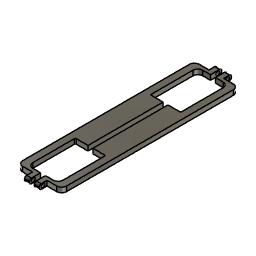
_Arm limb 1.2eed6a4d-bf02-4668-9319-046f86bff51b (Autodesk Fusion 360 design; units mm, degrees)
Autodesk Fusion 360 part; units mm, degrees
sketch "Sketch1" plane through (0, 0, 0) normal (0, 0, 1) x (1, 0, 0)
  line L0 (20, -90.5) -> (-20, -90.5)
  line L1 (-20, -90.5) -> (-20, 90.5)
  line L2 (-20, 90.5) -> (20, 90.5)
  line L3 (20, 90.5) -> (20, -90.5)
  line L4 (20, -90.5) -> (-20, 90.5) construction
  line L5 (-20, -90.5) -> (20, 90.5) construction
  dimension "d1" = 40
  dimension "d2" = 181
  constraint horizontal L0
  constraint perpendicular L0 L1
  constraint parallel L0 L2
  constraint parallel L1 L3
  constraint coincident L4 origin
  constraint coincident L5 origin
  measures "d1" distance of L1.end L2.end
  measures "d2" distance of L0.end L1.end
extrude "Extrude1" add sketch "Sketch1" along normal blind 5 makes body 1
sketch "Sketch2" plane through (0, 0, 5) normal (0, 0, 1) x (-1, 0, 0)
  line L0 (-20, -90.5) -> (20, -90.5)
  line L1 (20, -90.5) -> (20, 90.5)
  line L2 (20, 90.5) -> (-20, 90.5)
  line L3 (-20, 90.5) -> (-20, -90.5)
  line L4 (13, -38.45) -> (-13, -38.45)
  line L5 (-13, -38.45) -> (-13, -87.05)
  line L6 (-13, -87.05) -> (13, -87.05)
  line L7 (13, -87.05) -> (13, -38.45)
  line L8 (13, -38.45) -> (-13, -87.05) construction
  line L9 (-13, -38.45) -> (13, -87.05) construction
  line L10 (-13, 87.05) -> (13, 87.05)
  line L11 (13, 87.05) -> (13, 38.45)
  line L12 (13, 38.45) -> (-13, 38.45)
  line L13 (-13, 38.45) -> (-13, 87.05)
  line L14 (-13, 87.05) -> (13, 38.45) construction
  line L15 (13, 87.05) -> (-13, 38.45) construction
  point P0 (0, -62.75)
  point P1 (0, 62.75)
  dimension "d5" = 26
  dimension "d6" = 48.6
  dimension "d7" = 26
  dimension "d8" = 48.6
  constraint horizontal L4
  constraint perpendicular L4 L5
  constraint parallel L4 L6
  constraint parallel L5 L7
  constraint coincident L8 P0
  constraint coincident L9 P0
  constraint horizontal L10
  constraint perpendicular L10 L11
  constraint parallel L10 L12
  constraint parallel L11 L13
  constraint coincident L14 P1
  constraint coincident L15 P1
  measures "d5" distance of L5.end L6.end
  measures "d6" distance of L4.end L5.end
  measures "d7" distance of L11.end L12.end
  measures "d8" distance of L10.end L11.end
extrude "Extrude2" cut sketch "Sketch2" against normal blind 10 contours L4 L5 L6 L7 | L10 L11 L12 L13 bodies 1
sketch "Sketch3" plane through (0, -90.5, 0) normal (0, -1, 0) x (1, 0, 0)
  line L0 (-20, 0) -> (20, 0)
  line L1 (20, 0) -> (20, 5)
  line L2 (20, 5) -> (-20, 5)
  line L3 (-20, 5) -> (-20, 0)
  line L4 (-5, 5) -> (5, 5)
  line L5 (5, 5) -> (5, 0)
  line L6 (5, 0) -> (-5, 0)
  line L7 (-5, 0) -> (-5, 5)
  constraint horizontal L4
  constraint vertical L5
  constraint horizontal L6
  constraint vertical L7
  constraint coincident L0 L5.end
  constraint coincident L2 L4.start
extrude "Extrude3" add sketch "Sketch3" along normal blind 8 contours L0 L2 L4 L5 L6 L7 bodies 1
sketch "Sketch4" plane through (0, 90.5, 0) normal (0, 1, 0) x (-1, 0, 0)
  line L0 (-20, 0) -> (20, 0)
  line L1 (20, 0) -> (20, 5)
  line L2 (20, 5) -> (-20, 5)
  line L3 (-20, 5) -> (-20, 0)
  line L4 (-5, 5) -> (5, 5)
  line L5 (5, 5) -> (5, 0)
  line L6 (5, 0) -> (-5, 0)
  line L7 (-5, 0) -> (-5, 5)
  constraint horizontal L4
  constraint vertical L5
  constraint horizontal L6
  constraint vertical L7
  constraint coincident L0 L5.end
  constraint coincident L2 L4.start
extrude "Extrude4" add sketch "Sketch4" along normal blind 8 contours L0 L2 L4 L5 L6 L7 bodies 1
sketch "Sketch5" plane through (5, 0, 0) normal (1, 0, 0) x (0, 1, 0)
  line L0 (90.5, 5) -> (90.5, 0)
  line L1 (90.5, 0) -> (98.5, 0)
  line L2 (98.5, 0) -> (98.5, 5)
  line L3 (98.5, 5) -> (90.5, 5)
  circle A0 centre (94.5, 2.5) radius 2
  dimension "d21" = 4
  measures "d21" diameter of A0
sketch "Sketch6" plane through (5, 0, 0) normal (1, 0, 0) x (0, 1, 0)
  line L0 (-90.5, 0) -> (-90.5, 5)
  line L1 (-90.5, 5) -> (-98.5, 5)
  line L2 (-98.5, 5) -> (-98.5, 0)
  line L3 (-98.5, 0) -> (-90.5, 0)
  circle A0 centre (-94.5, 2.5) radius 2
  dimension "d22" = 4
  measures "d22" diameter of A0
extrude "Extrude5" cut sketch "Sketch5" sketch "Sketch6" against normal blind 15 contours A0 of sketch 2 contours A0 bodies 1
fillet "Fillet1" radius 5 4 edges at (-20, 90.5, 2.5) (20, 90.5, 2.5) (20, -90.5, 2.5) (-20, -90.5, 2.5) on bodies 1
fillet "Fillet2" radius 5 4 edges at (-13, 87.05, 2.5) (13, 87.05, 2.5) (13, -87.05, 2.5) (-13, -87.05, 2.5) on bodies 1
fillet "Fillet3" radius 1 4 edges at (-13, -38.45, 2.5) (13, -38.45, 2.5) (13, 38.45, 2.5) (-13, 38.45, 2.5) on bodies 1
fillet "Fillet4" radius 2 4 edges at (0, -98.5, 5) (0, -98.5, 0) (0, 98.5, 5) (0, 98.5, 0) on bodies 1
split "Split1" by plane through (0, 0, 0) normal (1, 0, 0) bodies 1 makes body 2 at (8, 12.8167, 5)
move_body "Move2" bodies 2 to x (1, 0, 0) y (0, 1, 0) z (0, 0, 1) at (5, 0, 0)
